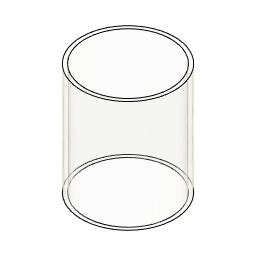
筒 (Autodesk Fusion 360 design; units mm, degrees)
Autodesk Fusion 360 part; units mm, degrees
sketch "スケッチ1" plane through (0, 0, 0) normal (0, 0, 1) x (1, 0, 0)
  circle A0 centre (0, 0) radius 25
  circle A1 centre (0, 0) radius 22.5
  dimension "d1" = 45
  constraint coincident A0.centre A1.centre
  constraint concentric A0 A1
  measures "d1" diameter of A1
extrude "押し出し1" add sketch "スケッチ1" along normal blind 70
sketch "スケッチ2" plane through (0, 0, 70) normal (0, 0, 1) x (-1, 0, 0)
  circle A0 centre (0, 0) radius 22.5
  circle A1 centre (0, 0) radius 25
  circle A2 centre (0, 0) radius 23
  constraint concentric A0 A2
extrude "押し出し2" cut sketch "スケッチ2" against normal blind 75 contours A2
extrude "押し出し3" cut 1 faces at (24.1546, -2.3847, 70) along direction (0, 0, -1) blind 10
